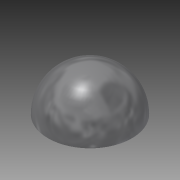
# Autodesk Inventor part: VR Camera Dome
Saved by Autodesk Inventor 2016 (Build 200138000, 138)
## iProperties
Created: 2016-10-29
Part Number: VR Camera Dome
Material: Generic
Document SubType Name: Modeling
Designer: eschr_000
Density: 1 g/cm^3
Appearance: Light Gray Reflective
Author: eschr_000
Autodesk Inventor part; units mm, degrees
ref_plane "YZ Plane" through (0, 0, 0) normal (1, 0, 0) x (0, 1, 0)
ref_plane "XZ Plane" through (0, 0, 0) normal (0, 1, 0) x (-1, 0, 0)
ref_plane "XY Plane" through (0, 0, 0) normal (0, 0, 1) x (1, 0, 0)
sketch "Sketch1" plane through (0, 0, 0) normal (1, 0, 0) x (0, 1, 0)
  line L0 (0, 0) -> (28, 0)
  line L1 (0, 0) -> (0, -28)
  line L2 (0, 0) -> (19.799, -19.799) construction
  arc A0 (0, -28) -> (28, 0) centre (0, 0) ccw
  dimension "d0" = 28
  dimension "d1" = 28
  dimension "d2" = 45
  dimension "d3" = 28
  constraints: 6 end point, 3 point on circle, 1 centre point, 1 horizontal, 1 vertical
  measures "d0" distance of L0.start L0.end
  measures "d1" distance of L0.start L1.end
  measures "d2" angle of L1 L2
  measures "d3" distance of L0.start L2.end
revolve "Revolution1" add sketch "Sketch1" angle 360 about axis through (0, 0, 0) along (0, 1, 0)
body "Solid1"
